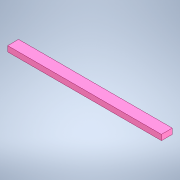
# Autodesk Inventor part: ledstrip
Saved by Autodesk Inventor 2021 (Build 250183000, 183)
## iProperties
Created: 2023-10-16
Part Number: ledstrip
Material: Generic
Document SubType Name: Modeling
Designer: Elias
Density: 1 g/cm^3
Appearance: Pink
Author: Elias
Autodesk Inventor part; units mm, degrees
ref_plane "YZ Plane" through (0, 0, 0) normal (1, 0, 0) x (0, 1, 0)
ref_plane "XZ Plane" through (0, 0, 0) normal (0, 1, 0) x (-1, 0, 0)
ref_plane "XY Plane" through (0, 0, 0) normal (0, 0, 1) x (1, 0, 0)
sketch "Sketch1" plane through (0, 0, 0) normal (1, 0, 0) x (0, 1, 0)
  line L0 (0, 0) -> (3, 0)
  line L1 (3, 0) -> (3, -6)
  line L2 (3, -6) -> (0, -6)
  line L3 (0, -6) -> (0, 0)
  dimension "d0" = 3
  dimension "d1" = 6
  constraints: 8 end point, 2 parallel, 1 horizontal, 1 perpendicular
  measures "d0" distance of L1.end L2.end
  measures "d1" distance of L0.end L1.end
extrude "Extrusion1" add sketch "Sketch1" along normal blind 85
body "Solid1"
